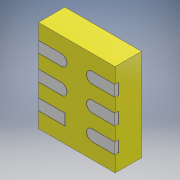
# Autodesk Inventor part: tsl2591
Saved by Autodesk Inventor 2017 (Build 210142000, 142)
## iProperties
Created: 2017-09-24
Part Number: tsl2591
Material: Generic
Document SubType Name: Modeling
Designer: P. Baesso
Density: 1 g/cm^3
Appearance: Default
Author: P. Baesso
Autodesk Inventor part; units mm, degrees
ref_plane "YZ Plane" through (0, 0, 0) normal (1, 0, 0) x (0, 1, 0)
ref_plane "XZ Plane" through (0, 0, 0) normal (0, 1, 0) x (-1, 0, 0)
ref_plane "XY Plane" through (0, 0, 0) normal (0, 0, 1) x (1, 0, 0)
sketch "Sketch1" plane through (0, 0, 0) normal (0, 1, 0) x (-1, 0, 0)
  line L0 (1, 1.2) -> (-1, 1.2)
  line L1 (-1, 1.2) -> (-1, -1.2)
  line L2 (-1, -1.2) -> (1, -1.2)
  line L3 (1, -1.2) -> (1, 1.2)
  line L4 (1, 1.2) -> (-1, -1.2) construction
  line L5 (-1, 1.2) -> (1, -1.2) construction
  line L6 (1, 0) -> (-1, 0) construction
  line L7 (0, -1.2) -> (0, 1.2) construction
  line L8 (1, -0.15) -> (0.4, -0.15)
  line L9 (0.25, 0) -> (0.25, 0)
  line L10 (0.4, 0.15) -> (1, 0.15)
  line L11 (1, 0.15) -> (1, -0.15)
  arc A0 (0.25, 0) -> (0.4, -0.15) centre (0.4, 0) ccw
  arc A1 (0.4, 0.15) -> (0.25, 0) centre (0.4, 0) ccw
  line L12 (-1, -0.15) -> (-0.4, -0.15)
  line L13 (-0.25, 0) -> (-0.25, 0)
  line L14 (-0.4, 0.15) -> (-1, 0.15)
  line L15 (-1, 0.15) -> (-1, -0.15)
  arc A2 (-0.4, -0.15) -> (-0.25, 0) centre (-0.4, 0) ccw
  arc A3 (-0.25, 0) -> (-0.4, 0.15) centre (-0.4, 0) ccw
  line L16 (1, -0.5) -> (0.3, -0.5)
  line L17 (0.3, -0.5) -> (0.3, -0.8)
  line L18 (0.3, -0.8) -> (1, -0.8)
  line L19 (1, -0.8) -> (1, -0.5)
  line L20 (1, 0.8) -> (0.4, 0.8)
  line L21 (0.25, 0.65) -> (0.25, 0.65)
  line L22 (0.4, 0.5) -> (1, 0.5)
  line L23 (1, 0.5) -> (1, 0.8)
  arc A4 (0.4, 0.8) -> (0.25, 0.65) centre (0.4, 0.65) ccw
  arc A5 (0.25, 0.65) -> (0.4, 0.5) centre (0.4, 0.65) ccw
  line L24 (-1, 0.8) -> (-0.4, 0.8)
  line L25 (-0.25, 0.65) -> (-0.25, 0.65)
  line L26 (-0.4, 0.5) -> (-1, 0.5)
  line L27 (-1, 0.5) -> (-1, 0.8)
  arc A6 (-0.25, 0.65) -> (-0.4, 0.8) centre (-0.4, 0.65) ccw
  arc A7 (-0.4, 0.5) -> (-0.25, 0.65) centre (-0.4, 0.65) ccw
  line L28 (-1, -0.8) -> (-0.4, -0.8)
  line L29 (-0.25, -0.65) -> (-0.25, -0.65)
  line L30 (-0.4, -0.5) -> (-1, -0.5)
  line L31 (-1, -0.5) -> (-1, -0.8)
  arc A8 (-0.25, -0.65) -> (-0.4, -0.5) centre (-0.4, -0.65) ccw
  arc A9 (-0.4, -0.8) -> (-0.25, -0.65) centre (-0.4, -0.65) ccw
  line L32 (0.4, 0.79) -> (0.99, 0.79)
  line L33 (0.99, 0.79) -> (0.99, 0.51)
  line L34 (0.99, 0.51) -> (0.4, 0.51)
  arc A10 (0.26, 0.65) -> (0.4, 0.51) centre (0.4, 0.65) ccw
  arc A11 (0.4, 0.79) -> (0.26, 0.65) centre (0.4, 0.65) ccw
  line L35 (-0.4, 0.79) -> (-0.99, 0.79)
  line L36 (-0.99, 0.79) -> (-0.99, 0.51)
  line L37 (-0.99, 0.51) -> (-0.4, 0.51)
  arc A12 (-0.4, 0.51) -> (-0.26, 0.65) centre (-0.4, 0.65) ccw
  arc A13 (-0.26, 0.65) -> (-0.4, 0.79) centre (-0.4, 0.65) ccw
  line L38 (-0.4, 0.14) -> (-0.99, 0.14)
  line L39 (-0.99, 0.14) -> (-0.99, -0.14)
  line L40 (-0.99, -0.14) -> (-0.4, -0.14)
  arc A14 (-0.4, -0.14) -> (-0.26, 0) centre (-0.4, 0) ccw
  arc A15 (-0.26, 0) -> (-0.4, 0.14) centre (-0.4, 0) ccw
  line L41 (-0.4, -0.51) -> (-0.99, -0.51)
  line L42 (-0.99, -0.51) -> (-0.99, -0.79)
  line L43 (-0.99, -0.79) -> (-0.4, -0.79)
  arc A16 (-0.4, -0.79) -> (-0.26, -0.65) centre (-0.4, -0.65) ccw
  arc A17 (-0.26, -0.65) -> (-0.4, -0.51) centre (-0.4, -0.65) ccw
  line L44 (0.31, -0.79) -> (0.31, -0.51)
  line L45 (0.31, -0.51) -> (0.99, -0.51)
  line L46 (0.99, -0.51) -> (0.99, -0.79)
  line L47 (0.99, -0.79) -> (0.31, -0.79)
  arc A18 (0.26, 0) -> (0.4, -0.14) centre (0.4, 0) ccw
  line L48 (0.4, -0.14) -> (0.99, -0.14)
  line L49 (0.99, -0.14) -> (0.99, 0.14)
  line L50 (0.99, 0.14) -> (0.4, 0.14)
  arc A19 (0.4, 0.14) -> (0.26, 0) centre (0.4, 0) ccw
  point P0 (0, 0)
  point P1 (0.25, 0.15)
  point P2 (0.25, -0.15)
  point P3 (-0.25, 0.15)
  point P4 (-0.25, -0.15)
  point P5 (0.25, 0.5)
  point P6 (0.25, 0.8)
  point P7 (-0.25, 0.5)
  point P8 (-0.25, 0.8)
  point P9 (-0.25, -0.5)
  point P10 (-0.25, -0.8)
  dimension "d0" = 2
  dimension "d1" = 2.4
  dimension "d2" = 0.75
  dimension "d3" = 0.3
  dimension "d4" = 0.15
  dimension "d5" = 0.7
  dimension "d6" = 0.3
  dimension "d7" = 0.65
  dimension "d8" = 0.75
  dimension "d9" = 0.3
  dimension "d10" = 0.65
  dimension "d11" = 0.15
  dimension "d12" = 0.75
  dimension "d13" = 0.3
  dimension "d14" = 0.15
  dimension "d15" = 0.65
  dimension "d16" = 0.01
  dimension "d17" = 0.01
  dimension "d18" = 0.01
  dimension "d19" = 0.01
  dimension "d20" = 0.01
  dimension "d21" = 0.01
  constraints: 102 end point, 40 point on circle, 24 point on line, 20 centre point, 20 symmetric about line, 15 parallel, 12 tangent, 6 midpoint, 6 perpendicular, 5 horizontal, 3 concentric, 28 other
  measures "d0" distance of L2.end L1.end
  measures "d1" distance of L1.end L0.end
  measures "d2" distance of point (0.25, 0.15) L10.end
  measures "d3" distance of point (0.25, -0.15) point (0.25, 0.15)
  measures "d4" radius of A0
  measures "d5" distance of L18.end L17.end
  measures "d6" distance of L17.end L16.end
  measures "d7" distance between parallel lines of L18 L8
  measures "d8" distance of L22.end point (0.25, 0.5)
  measures "d9" distance of point (0.25, 0.5) point (0.25, 0.8)
  measures "d10" distance between parallel lines of L8 L22
  measures "d11" radius of A4
  measures "d12" distance of L30.end point (-0.25, -0.5)
  measures "d13" distance of point (-0.25, -0.5) point (-0.25, -0.8)
  measures "d14" radius of A8
  measures "d15" distance between parallel lines of L28 L12
  measures "d16" distance between parallel lines of L20 L32
  measures "d17" radial gap between concentric circles of A6 A13
  measures "d18" radial gap between concentric circles of A3 A15
  measures "d19" radial gap between concentric circles of A8 A17
  measures "d20" distance between parallel lines of L17 L44
  measures "d21" radial gap between concentric circles of A1 A19
extrude "Extrusion1" add sketch "Sketch1" along normal blind 0.097 contours L32 L33 L34 A10 A11 | A13 A12 L37 L36 L35 | A15 A14 L40 L39 L38 | A17 A16 L43 L42 L41 | L44 L45 L46 L47 | A19 L50 L49 L48 A18
extrude "Extrusion2" add sketch "Sketch1" along normal blind 0.097 contours L3 L20 A4 A5 L22 L10 A1 A0 L8 L16 L17 L18 L2 L1 L28 A9 A8 L30 L12 A2 A3 L14 L26 A7 A6 L24 L0
sketch "Sketch2" plane through (0, 0.097, 0) normal (0, 1, 0) x (1, 0, 0)
  line L0 (1, -1.2) -> (1, -0.8) projected
  line L1 (-1, 1.2) -> (1, 1.2)
  line L2 (1, 1.2) -> (1, -1.2)
  line L3 (1, -1.2) -> (-1, -1.2)
  line L4 (-1, -1.2) -> (-1, 1.2)
  point P0 (0, 0)
  constraints: 8 end point, 2 parallel, 1 horizontal, 1 perpendicular
extrude "Extrusion3" add sketch "Sketch2" along normal blind 0.258
sketch "Sketch3" plane through (0, 0.355, 0) normal (0, 1, 0) x (1, 0, 0)
  line L0 (-0.401, 0) -> (0.401, 0)
  line L1 (0.401, 0) -> (0.401, -0.716)
  line L2 (0.401, -0.716) -> (-0.401, -0.716)
  line L3 (-0.401, -0.716) -> (-0.401, 0)
  line L4 (-1, -0.15) -> (-1, 0.15) construction
  line L5 (-1, 0) -> (0.9997, 0) construction
  line L6 (1, 1.2) -> (-1, 1.2) construction
  line L7 (0, 1.2) -> (0, -1.2) construction
  line L8 (-1, -1.2) -> (1, -1.2) construction
  point P0 (0, 0)
  dimension "d46" = 0.802
  dimension "d47" = 0.716
  constraints: 12 end point, 3 midpoint, 2 horizontal, 2 parallel, 1 collinear, 1 perpendicular, 1 other
  measures "d46" distance of L1.end L2.end
  measures "d47" distance of L0.end L1.end
extrude "Extrusion4" add sketch "Sketch3" along normal blind 0.05
sketch "Sketch4" plane through (0, 0.355, 0) normal (0, 1, 0) x (1, 0, 0)
  line L0 (-1, 1.2) -> (-1, -1.2) projected
  line L1 (-1, -1.2) -> (1, -1.2) projected
  line L2 (-1, 1.2) -> (1, 1.2)
  line L3 (1, 1.2) -> (1, -1.2)
  line L4 (1, -1.2) -> (-1, -1.2)
  line L5 (-1, -1.2) -> (-1, 1.2)
  line L6 (0.401, 0) -> (-0.401, 0) projected
  line L7 (-0.401, 0) -> (-0.401, -0.716) projected
  line L8 (-0.401, -0.716) -> (0.401, -0.716) projected
  line L9 (0.401, -0.716) -> (0.401, 0) projected
  line L10 (-0.411, 0.01) -> (0.411, 0.01)
  line L11 (0.411, 0.01) -> (0.411, -0.726)
  line L12 (0.411, -0.726) -> (-0.411, -0.726)
  line L13 (-0.411, -0.726) -> (-0.411, 0.01)
  point P0 (0, 0)
  dimension "d50" = 0.01
  constraints: 16 end point, 2 parallel, 1 horizontal, 1 perpendicular, 3 other
  measures "d50" distance between parallel lines of L6 L10
extrude "Extrusion5" add sketch "Sketch4" along normal up to surface (0.05 mm away) contours L2 L3 L1 L0
sketch "Sketch5" plane through (-1, 0.405, -1.2) normal (0, 1, 0) x (1, 0, 0)
  line L0 (0, 0) -> (0, -0.4) projected
  line L1 (2, 0) -> (2, -2.4) projected
  line L2 (0, 0) -> (2, 0)
  line L3 (2, 0) -> (2, -2.4)
  line L4 (2, -2.4) -> (0, -2.4)
  line L5 (0, -2.4) -> (0, 0)
  point P0 (1, -1.2)
  constraints: 8 end point, 2 parallel, 1 horizontal, 1 perpendicular
extrude "Extrusion6" add sketch "Sketch5" along normal blind 0.285
body "Solid1"
